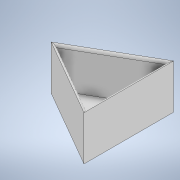
# Autodesk Inventor part: TrojkatP
Saved by Autodesk Inventor 2020.3 (Build 243373000, 373)
## iProperties
Created: 2021-05-21
Part Number: TrojkatP
Material: Generic
Document SubType Name: Modeling
Designer: patry
Density: 1 g/cm^3
Appearance: Default
Author: patry
Autodesk Inventor part; units mm, degrees
ref_plane "YZ Plane" through (0, 0, 0) normal (1, 0, 0) x (0, 1, 0)
ref_plane "XZ Plane" through (0, 0, 0) normal (0, 1, 0) x (-1, 0, 0)
ref_plane "XY Plane" through (0, 0, 0) normal (0, 0, 1) x (1, 0, 0)
sketch "Sketch1" plane through (0, 0, 0) normal (0, 1, 0) x (-1, 0, 0)
  circle A0 centre (0, 0) radius 52.5
  line L0 (0, 0) -> (52.5, 0)
  line L1 (52.5, 0) -> (0, 0)
  line L2 (52.5, 0) -> (0, 0)
  line L3 (0, 0) -> (-26.25, 0)
  line L4 (-26.25, 0) -> (-26.25, 45.4663)
  line L5 (52.5, 0) -> (-26.25, 45.4663)
  line L6 (-26.25, 0) -> (-26.25, -45.4663)
  line L7 (52.5, 0) -> (-26.25, -45.4663)
  constraints: 16 end point, 3 point on circle, 2 horizontal, 2 point on line, 1 centre point, 1 coincident, 1 collinear, 1 perpendicular
extrude "Extrusion1" add sketch "Sketch1" along normal blind 5 contours L7 L6 L3 L0 | L0 L3 L4 L5
sketch "Sketch5" plane through (0, 5, 0) normal (0, 1, 0) x (1, 0, 0)
  circle A0 centre (0, 0) radius 4.25
  dimension "d9" = 8.5
  constraints: 1 centre point, 1 coincident
  measures "d9" diameter of A0
extrude "Extrusion3" cut sketch "Sketch5" against normal blind 2
sketch "Sketch6" plane through (0, 5, 0) normal (0, 1, 0) x (1, 0, 0)
  circle A0 centre (0, 0) radius 2.5
  dimension "d12" = 5
  constraints: 1 centre point, 1 coincident
  measures "d12" diameter of A0
extrude "Extrusion4" add sketch "Sketch6" against normal blind 10
sketch "Sketch7" plane through (0, 5, 0) normal (0, 1, 0) x (1, 0, 0)
  circle A0 centre (0, 0) radius 4.25 projected
  circle A1 centre (0, 0) radius 2.5
  constraints: 1 centre point, 1 coincident
extrude "Extrusion5" cut sketch "Sketch7" against normal through all contours A1
sketch "Sketch8" plane through (0, 5, 0) normal (0, 1, 0) x (1, 0, 0)
  line L0 (-52.5, 0) -> (26.25, -45.4663) projected
  line L1 (-52.5, 0) -> (26.25, -45.4663)
  line L2 (26.25, 45.4663) -> (-52.5, 0) projected
  line L3 (26.25, -45.4663) -> (26.25, 45.4663)
  line L4 (26.25, 45.4663) -> (-52.5, 0)
  line L5 (26.25, -45.4663) -> (26.25, 45.4663) projected
  line L6 (26.25, 0) -> (23.75, 0)
  line L7 (-13.125, -22.7332) -> (-11.875, -20.5681)
  line L8 (-13.125, 22.7332) -> (-11.875, 20.5681)
  line L9 (-11.875, -20.5681) -> (-47.5, 0)
  line L10 (-47.5, 0) -> (-11.875, 20.5681)
  line L11 (23.75, 0) -> (23.75, 41.1362)
  line L12 (23.75, 41.1362) -> (-11.875, 20.5681)
  line L13 (23.75, 0) -> (23.75, -41.1362)
  line L14 (-11.875, -20.5681) -> (23.75, -41.1362)
  point P0 (0, 0)
  dimension "d17" = 2.5
  dimension "d18" = 2.5
  constraints: 24 end point, 3 midpoint, 3 parallel, 3 point on line, 2 perpendicular, 2 vertical, 1 collinear, 1 horizontal
  measures "d17" distance of L6.start L6.end
  measures "d18" distance of L7.start L7.end
extrude "Extrusion6" add sketch "Sketch8" along normal blind 40 contours L2 L8 L10 L9 L7 L0 | L7 L14 L13 L6 L3 L0 | L2 L3 L6 L11 L12 L8
fillet "Fillet1" radius 2.5 3 edges at (-11.875, 45, -20.5681) (23.75, 45, 0) (-11.875, 45, 20.5681)
body "Solid1"
